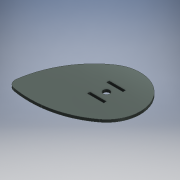
# Autodesk Inventor part: leva00
Saved by Autodesk Inventor 2016 (Build 200138000, 138)
## iProperties
Created: 2016-09-20
Part Number: leva00
Material: Madera (abedul)
Document SubType Name: Modeling
Designer: i95sa
Density: 0.55 g/cm^3
Appearance: Gris plomo - Pulido
Author: i95sa
Autodesk Inventor part; units mm, degrees
ref_plane "YZ Plane" through (0, 0, 0) normal (1, 0, 0) x (0, 1, 0)
ref_plane "XZ Plane" through (0, 0, 0) normal (0, 1, 0) x (-1, 0, 0)
ref_plane "XY Plane" through (0, 0, 0) normal (0, 0, 1) x (1, 0, 0)
sketch "Boceto1" plane through (0, 0, 0) normal (0, 0, 1) x (1, 0, 0)
  arc A0 (41.543, 30.1828) -> (-41.543, -30.1828) centre (0, 0) ccw
  arc A1 (-63.9314, -46.4489) -> (-83.1051, -60.3794) centre (-73.5183, -53.4142) ccw
  line L0 (-85.8808, -62.396) -> (-92.846, -52.8092)
  line L1 (-29.6885, 41.8976) -> (-41.2973, 57.8757)
  line L2 (-41.2973, 57.8757) -> (-92.846, -52.8092)
  line L3 (-92.846, -52.8092) -> (-72.8345, -9.8406)
  arc A2 (-29.6885, 41.8976) -> (-72.8345, -9.8406) centre (46.2832, -65.3167) ccw
  arc A3 (-72.8345, -9.8406) -> (-85.2521, -51.7589) centre (61.6763, -72.4857) ccw
  line L4 (3.1956, 2.3218) -> (41.543, 30.1828)
  line L5 (-3.1956, -2.3218) -> (-85.8808, -62.396)
  arc A4 (-41.543, -30.1828) -> (41.543, 30.1828) centre (0, 0) ccw
  arc A5 (-83.1051, -60.3794) -> (-63.9314, -46.4489) centre (-73.5183, -53.4142) ccw
  line L6 (-85.8808, -62.396) -> (-78.9155, -71.9829)
  line L7 (30.6728, -41.1826) -> (42.2815, -57.1607)
  line L8 (42.2815, -57.1607) -> (-78.9155, -71.9829)
  line L9 (-78.9155, -71.9829) -> (-31.8661, -66.2288)
  arc A6 (-31.8661, -66.2288) -> (30.6728, -41.1826) centre (-47.8176, 64.2019) ccw
  arc A7 (-75.57, -65.0852) -> (-31.8661, -66.2288) centre (-49.8789, 81.057) ccw
  dimension "d0" = 102.7
  dimension "d6" = 23.7
  dimension "d7" = 11.85
  dimension "d8" = 19.75
  dimension "d9" = 47.4
  constraints: 20 end point, 20 point on circle, 8 centre point, 6 symmetric about line, 5 point on line, 4 tangent, 1 collinear, 4 other
  measures "d0" diameter of A0
  measures "d6" diameter of A1
  measures "d7" distance of L0.start L0.end
  measures "d8" distance of L1.start L1.end
  measures "d9" distance of L0.end L3.end
extrude "Extrusión2" add sketch "Boceto1" along normal blind 4 contours A4 A0 | A0 L5 A1 A3 A2 | A6 A7 A5 L5 A4 | L5 A1 | A5 L5
sketch "Boceto2" plane through (0, 0, 4) normal (0, 0, 1) x (1, 0, 0)
  line L0 (0, 0) -> (0, 12.5)
  line L1 (0, 12.5) -> (-12.5, 12.5)
  line L2 (-12.5, 12.5) -> (-12.5, 16.7)
  line L3 (-12.5, 16.7) -> (12.5, 16.7)
  line L4 (12.5, 16.7) -> (12.5, 12.5)
  line L5 (12.5, 12.5) -> (0, 12.5)
  line L6 (0, 0) -> (12.5, 0)
  line L7 (0, 0) -> (0, -12.5)
  line L8 (0, -12.5) -> (-12.5, -12.5)
  line L9 (-12.5, -12.5) -> (-12.5, -16.7)
  line L10 (-12.5, -16.7) -> (12.5, -16.7)
  line L11 (12.5, -16.7) -> (12.5, -12.5)
  line L12 (12.5, -12.5) -> (0, -12.5)
  circle A0 centre (0, 0) radius 5
  dimension "d24" = 12.5
  dimension "d25" = 12.5
  dimension "d26" = 4.2
  dimension "d27" = 25
  dimension "d28" = 10
  constraints: 26 end point, 5 perpendicular, 5 symmetric about line, 3 point on line, 1 centre point, 1 coincident, 1 parallel, 1 vertical
  measures "d24" distance of L0.start L0.end
  measures "d25" distance of L0.end L1.end
  measures "d26" distance of L1.end L2.end
  measures "d27" distance of L2.end L3.end
  measures "d28" diameter of A0
extrude "Extrusión3" cut sketch "Boceto2" against normal blind 4
